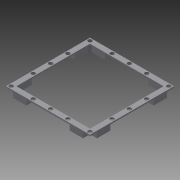
# Autodesk Inventor part: Base
Saved by Autodesk Inventor 2014 SP1 (Build 180222100, 222)
## iProperties
Created: 2015-03-29
Part Number: Base
Material: ABS Plastic
Document SubType Name: Modeling
Designer: Erin
Density: 1.06 g/cm^3
Appearance: Smooth - White
Mass: 7.68531 g
Surface Area: 72.7035 cm^2
Volume: 7.2503 cm^3
Author: Erin
Autodesk Inventor part; units mm, degrees
ref_plane "YZ Plane" through (0, 0, 0) normal (1, 0, 0) x (0, 1, 0)
ref_plane "XZ Plane" through (0, 0, 0) normal (0, 1, 0) x (-1, 0, 0)
ref_plane "XY Plane" through (0, 0, 0) normal (0, 0, 1) x (1, 0, 0)
sketch "Sketch1" plane through (0, 0, 0) normal (0, 0, 1) x (1, 0, 0)
  line L0 (-48, 48) -> (48, 48)
  line L1 (48, 48) -> (48, -48)
  line L2 (48, -48) -> (-48, -48)
  line L3 (-48, -48) -> (-48, 48)
  line L4 (42, 42) -> (-42, 42)
  line L5 (-42, 42) -> (-42, -42)
  line L6 (-42, -42) -> (42, -42)
  line L7 (42, -42) -> (42, 42)
  line L8 (0, 152.7233) -> (0, -72.1628) construction
  line L9 (-77.8847, 0) -> (88.8171, 0) construction
  line L10 (-48, 45) -> (48, 45) construction
  circle A0 centre (0, 45) radius 2.25
  circle A1 centre (-19.75, 45) radius 2.25
  circle A2 centre (19.75, 45) radius 2.25
  line L11 (-45, 48) -> (-45, -48) construction
  circle A3 centre (-45, 45) radius 2.25
  circle A4 centre (-45, 0) radius 2.25
  line L12 (-48, -45) -> (48, -45) construction
  circle A5 centre (-45, -45) radius 2.25
  circle A6 centre (-45, 19.75) radius 2.25
  circle A7 centre (-45, -19.75) radius 2.25
  point P0 (0, 0)
  point P1 (0, 48)
  point P2 (48, 0)
  dimension "d0" = 96
  dimension "d1" = 96
  dimension "d2" = 6
  dimension "d5" = 3
  dimension "d6" = 4.5
  dimension "d7" = 4.5
  dimension "d8" = 4.5
  dimension "d9" = 22
  dimension "d10" = 22
  dimension "d11" = 3
  dimension "d12" = 4.5
  dimension "d13" = 4.5
  dimension "d14" = 3
  dimension "d15" = 4.5
  dimension "d31" = 4.5
  dimension "d32" = 4.5
  dimension "d33" = 22
  dimension "d34" = 22
  constraints: 26 end point, 14 point on line, 8 centre point, 6 perpendicular, 5 parallel, 4 midpoint, 2 horizontal, 1 horizontal alignment, 1 vertical, 1 vertical alignment, 3 other
  measures "d0" distance of L1.end L2.end
  measures "d1" distance of L0.end L1.end
  measures "d2" distance between parallel lines of L4 L0
  measures "d5" distance between parallel lines of L10 L0
  measures "d6" diameter of A0
  measures "d7" diameter of A1
  measures "d8" diameter of A2
  measures "d11" distance between parallel lines of L11 L3
  measures "d12" diameter of A3
  measures "d13" diameter of A4
  measures "d14" distance between parallel lines of L12 L2
  measures "d15" diameter of A5
  measures "d31" diameter of A6
  measures "d32" diameter of A7
extrude "Extrusion1" add sketch "Sketch1" along normal blind 1.5 contours L0 L1 L2 L3 | A0 | A1 | A2 | A3 | A4 | A5 | A6 | A7
extrude "Extrusion2" cut sketch "Sketch1" along normal blind 10 contours A0 | A1 | A2
mirror "Mirror1" about plane through (0, 0, 0) normal (0, 1, 0) of "Extrusion2"
extrude "Extrusion3" cut sketch "Sketch1" along normal blind 10 contours A3 | A4 | A5 | A6 | A7
mirror "Mirror2" about plane through (0, 0, 0) normal (1, 0, 0) of "Extrusion3"
sketch "Sketch2" plane through (0, 0, 0) normal (0, 0, -1) x (-1, 0, 0)
  circle A0 centre (-45, 19.75) radius 2.25 projected
  circle A1 centre (-45, 0) radius 2.25 projected
  circle A2 centre (-45, 45) radius 2.25 projected
  circle A3 centre (0, 45) radius 2.25 projected
  circle A4 centre (-19.75, 45) radius 2.25 projected
  line L0 (48, 48) -> (-48, 48) projected
  line L1 (-48, 48) -> (-48, -48) projected
  line L2 (-42, -42) -> (-42, 42) projected
  line L3 (-42, 42) -> (42, 42) projected
  line L4 (-48, 40) -> (-42, 40)
  line L5 (-42, 40) -> (-42, 24.75)
  line L6 (-42, 24.75) -> (-48, 24.75)
  line L7 (-48, 24.75) -> (-48, 40)
  line L8 (-48, 14.75) -> (-42, 14.75)
  line L9 (-42, 14.75) -> (-42, 5)
  line L10 (-42, 5) -> (-48, 5)
  line L11 (-48, 5) -> (-48, 14.75)
  line L12 (-40, 48) -> (-24.75, 48)
  line L13 (-24.75, 48) -> (-24.75, 42)
  line L14 (-24.75, 42) -> (-40, 42)
  line L15 (-40, 42) -> (-40, 48)
  line L16 (-14.75, 48) -> (-5, 48)
  line L17 (-5, 48) -> (-5, 42)
  line L18 (-5, 42) -> (-14.75, 42)
  line L19 (-14.75, 42) -> (-14.75, 48)
  dimension "d35" = 5
  dimension "d36" = 5
  dimension "d37" = 5
  dimension "d38" = 5
  dimension "d39" = 5
  dimension "d40" = 5
  dimension "d41" = 5
  dimension "d42" = 5
  constraints: 32 end point, 8 parallel, 4 collinear, 4 horizontal, 4 perpendicular, 4 point on line
  measures "d35" distance from line of A2.centre L4
  measures "d36" distance from line of A0.centre L6
  measures "d37" distance from line of L8 A0.centre
  measures "d38" distance from line of A1.centre L10
  measures "d39" distance from line of A2.centre L15
  measures "d40" distance from line of A4.centre L13
  measures "d41" distance from line of A4.centre L19
  measures "d42" distance from line of A3.centre L17
extrude "Extrusion4" add sketch "Sketch2" along normal blind 6 contours L13 L3 L15 L0 | L4 L2 L6 L1
mirror "Mirror3" about plane through (0, 0, 0) normal (1, 0, 0) of "Extrusion4"
mirror "Mirror4" about plane through (0, 0, 0) normal (0, 1, 0) of "Extrusion4", "Mirror3"
body "Solid1"
